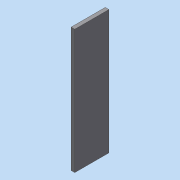
# Autodesk Inventor part: Bearing-Side
Saved by Autodesk Inventor 2016 SP1 (Build 200210100, 210)
## iProperties
Created: 2016-03-02
Part Number: Bearing-Side
Material: Generic
Document SubType Name: Modeling
Designer: Mohamed A.
Density: 1 g/cm^3
Appearance: Default
Author: Mohamed A.
Autodesk Inventor part; units mm, degrees
ref_plane "YZ Plane" through (0, 0, 0) normal (1, 0, 0) x (0, 1, 0)
ref_plane "XZ Plane" through (0, 0, 0) normal (0, 1, 0) x (-1, 0, 0)
ref_plane "XY Plane" through (0, 0, 0) normal (0, 0, 1) x (1, 0, 0)
sketch "Sketch2" plane through (0, 0, 0) normal (1, 0, 0) x (0, 1, 0)
  line L0 (12.5, -51) -> (-12.5, -51)
  line L1 (-12.5, -51) -> (-12.5, 51)
  line L2 (-12.5, 51) -> (12.5, 51)
  line L3 (12.5, 51) -> (12.5, -51)
  line L4 (12.5, -51) -> (-12.5, 51) construction
  line L5 (-12.5, -51) -> (12.5, 51) construction
  line L6 (-12.5, 51) -> (-15.5, 51)
  line L7 (-15.5, 51) -> (-15.5, -51)
  line L8 (-15.5, -51) -> (-12.5, -51)
  point P0 (0, 0)
  dimension "d0" = 25
  dimension "d1" = 102
  dimension "d4" = 3
  constraints: 18 end point, 4 perpendicular, 2 midpoint, 2 parallel, 1 horizontal
  measures "d0" distance of L1.end L2.end
  measures "d1" distance of L0.end L1.end
  measures "d4" distance of L1.end L6.end
extrude "Extrusion1" add sketch "Sketch2" along normal blind 3
body "Solid1"
